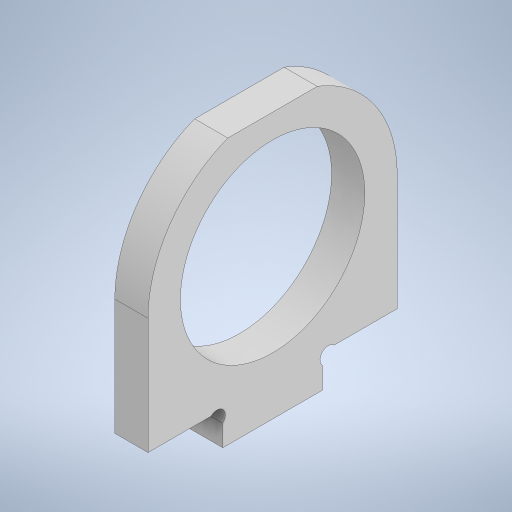
# Autodesk Inventor part: Motor Mount
Saved by Autodesk Inventor 2023 (Build 270158000, 158)
## iProperties
Created: 2023-01-08
Part Number: Motor Mount
Material: Generic
Document SubType Name: Modeling
Designer: justi
Density: 1 g/cm^3
Appearance: Default
Author: justi
Autodesk Inventor part; units mm, degrees
ref_plane "YZ Plane" through (0, 0, 0) normal (1, 0, 0) x (0, 1, 0)
ref_plane "XZ Plane" through (0, 0, 0) normal (0, 1, 0) x (-1, 0, 0)
ref_plane "XY Plane" through (0, 0, 0) normal (0, 0, 1) x (1, 0, 0)
sketch "Sketch1" plane through (0, 0, 0) normal (1, 0, 0) x (0, 1, 0)
  line L0 (0, 0) -> (88.9, 0)
  line L1 (88.9, 0) -> (88.9, -95.25)
  line L2 (88.9, -95.25) -> (0, -95.25)
  line L3 (0, -95.25) -> (0, 0)
  line L4 (0, -28.575) -> (-12.7, -28.575)
  line L5 (-12.7, -28.575) -> (-12.7, -66.675)
  line L6 (-12.7, -66.675) -> (0, -66.675)
  line L7 (0, -66.675) -> (0, -28.575)
  circle A0 centre (44.45, -47.625) radius 47.625
  circle A1 centre (44.45, -47.625) radius 35.2425
  point P0 (-12.7, -47.625)
  point P1 (0, -66.675)
  point P2 (44.45, -95.25)
  point P3 (88.9, -64.7229)
  point P4 (88.9, -30.5271)
  point P5 (44.45, 0)
  dimension "d0" = 88.9
  dimension "d1" = 95.25
  dimension "d2" = 12.7
  dimension "d3" = 38.1
  dimension "d4" = 47.625
  dimension "d5" = 95.25
  dimension "d6" = 70.485
  constraints: 16 end point, 4 parallel, 2 centre point, 2 horizontal, 2 perpendicular, 1 coincident, 1 midpoint, 1 point on line
  measures "d0" distance of L1.end L2.end
  measures "d1" distance of L0.end L1.end
  measures "d2" distance of L6.end L5.end
  measures "d3" distance of L4.end L5.end
  measures "d4" vertical distance of L0.start point (-12.7, -47.625)
  measures "d5" diameter of A0
  measures "d6" diameter of A1
extrude "Extrusion1" add sketch "Sketch1" along normal blind 12.7 contours L0 A0 L3 | A0 L1 L3 | L3 A0 L6 L5 L4 | L3 A0 | A0 L2 L3
sketch "Sketch2" plane through (12.7, 0, 0) normal (1, 0, 0) x (0, 0, -1)
  line L0 (28.575, 0) -> (28.575, -12.7) projected
  line L1 (28.575, 0) -> (26.3299, -2.2451)
  line L2 (66.675, -12.7) -> (66.675, 0) projected
  line L3 (66.675, 0) -> (68.9201, -2.2451)
  line L4 (66.675, 0) -> (95.25, 0) projected
  circle A0 centre (68.9201, -2.2451) radius 3.175
  circle A1 centre (26.3299, -2.2451) radius 3.175
  point P0 (0, 0)
  dimension "d9" = 3.175
  dimension "d10" = 45
  dimension "d11" = 3.175
  dimension "d12" = 45
  dimension "d13" = 6.35
  dimension "d14" = 6.35
  constraints: 4 end point, 2 centre point, 1 point on line
  measures "d9" distance of L0.start L1.end
  measures "d10" angle of L0 L1
  measures "d11" distance of L2.end L3.end
  measures "d12" angle of L4 L3
  measures "d13" diameter of A0
  measures "d14" diameter of A1
extrude "Extrusion2" cut sketch "Sketch2" against normal blind 12.7
body "Solid1"
